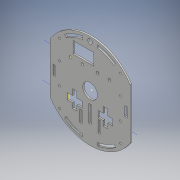
# Autodesk Inventor part: base_quick
Saved by Autodesk Inventor 2017.2 (Build 212233000, 233)
## iProperties
Created: 2017-07-13
Part Number: base_quick
Material: Generic
Document SubType Name: Modeling
Designer: Nic
Density: 1 g/cm^3
Appearance: Default
Author: Nic
Autodesk Inventor part; units mm, degrees
ref_plane "YZ Plane" through (0, 0, 0) normal (1, 0, 0) x (0, 1, 0)
ref_plane "XZ Plane" through (0, 0, 0) normal (0, 1, 0) x (-1, 0, 0)
ref_plane "XY Plane" through (0, 0, 0) normal (0, 0, 1) x (1, 0, 0)
sketch "Sketch1" plane through (0, 0, 0) normal (0, 1, 0) x (-1, 0, 0)
  line L0 (42.2, 26.8172) -> (42.2, -26.8172)
  line L1 (0, 0) -> (0, -50) construction
  line L2 (-42.2, 26.8172) -> (-42.2, -26.8172)
  arc A0 (42.2, 26.8172) -> (-42.2, 26.8172) centre (0, 0) ccw
  arc A1 (-42.2, -26.8172) -> (42.2, -26.8172) centre (0, 0) ccw
  line L3 (39.2, 5) -> (36.7, 5)
  line L4 (36.7, 5) -> (36.7, -5)
  line L5 (36.7, -5) -> (39.2, -5)
  line L6 (39.2, -5) -> (39.2, 5)
  circle A2 centre (0, 0) radius 7.75
  line L7 (1.25, -12) -> (-1.25, -12)
  line L8 (-1.25, -12) -> (-1.25, -30)
  line L9 (-1.25, -30) -> (1.25, -30)
  line L10 (1.25, -30) -> (1.25, -12)
  line L11 (10.95, -22) -> (8.45, -22)
  line L12 (8.45, -22) -> (8.45, -34)
  line L13 (8.45, -34) -> (10.95, -34)
  line L14 (10.95, -34) -> (10.95, -22)
  line L15 (8.45, -13.6) -> (8.45, -20)
  line L16 (24.05, -20) -> (24.05, -13.6)
  line L17 (18.55, -7.2) -> (13.95, -7.2)
  line L18 (13.95, -25.2) -> (18.55, -25.2)
  line L19 (18, 37.1) -> (-4, 37.1)
  line L20 (-4, 37.1) -> (-4, 24.85)
  line L21 (-4, 24.85) -> (18, 24.85)
  line L22 (18, 24.85) -> (18, 37.1)
  line L23 (25.2374, 36.0427) -> (26.9581, 38.5001)
  line L24 (0, 0) -> (7.6405, 43.3315) construction
  line L25 (7.6405, 43.3315) -> (8.1615, 46.286)
  line L26 (0, 0) -> (42.2, 0) construction
  line L27 (25.2374, -36.0427) -> (26.9581, -38.5001)
  line L28 (7.6405, -43.3315) -> (8.1615, -46.286)
  arc A3 (7.6405, -43.3315) -> (25.2374, -36.0427) centre (0, 0) ccw
  arc A4 (25.2374, 36.0427) -> (7.6405, 43.3315) centre (0, 0) ccw
  arc A5 (8.1615, -46.286) -> (26.9581, -38.5001) centre (0, 0) ccw
  arc A6 (26.9581, 38.5001) -> (8.1615, 46.286) centre (0, 0) ccw
  line L29 (0, 0) -> (25.2374, 36.0427) construction
  line L30 (16.25, -7.2) -> (16.25, -25.2) construction
  line L31 (18.55, -25.2) -> (18.55, -20)
  line L32 (18.55, -13.6) -> (18.55, -7.2)
  line L33 (24.05, -13.6) -> (18.55, -13.6)
  line L34 (13.95, -13.6) -> (8.45, -13.6)
  line L35 (13.95, -7.2) -> (13.95, -13.6)
  line L36 (13.95, -20) -> (13.95, -25.2)
  line L37 (8.45, -20) -> (13.95, -20)
  line L38 (18.55, -20) -> (24.05, -20)
  line L39 (-39.2, 5) -> (-36.7, 5)
  line L40 (-36.7, 5) -> (-36.7, -5)
  line L41 (-36.7, -5) -> (-39.2, -5)
  line L42 (-39.2, -5) -> (-39.2, 5)
  line L43 (-8.45, 16.1) -> (-8.45, 9.2)
  line L44 (-11.55, 9.2) -> (-11.55, 16.1)
  line L45 (-10.95, -22) -> (-8.45, -22)
  line L46 (-8.45, -22) -> (-8.45, -34)
  line L47 (-8.45, -34) -> (-10.95, -34)
  line L48 (-10.95, -34) -> (-10.95, -22)
  line L49 (-8.45, -13.6) -> (-8.45, -20)
  line L50 (-24.05, -20) -> (-24.05, -13.6)
  line L51 (-18.55, -7.2) -> (-13.95, -7.2)
  line L52 (-13.95, -25.2) -> (-18.55, -25.2)
  line L53 (-25.2374, 36.0427) -> (-26.9581, 38.5001)
  line L54 (-7.6405, 43.3315) -> (-8.1615, 46.286)
  line L55 (0, 0) -> (-42.2, 0) construction
  line L56 (-25.2374, -36.0427) -> (-26.9581, -38.5001)
  line L57 (-7.6405, -43.3315) -> (-8.1615, -46.286)
  arc A7 (-25.2374, -36.0427) -> (-7.6405, -43.3315) centre (0, 0) ccw
  arc A8 (-7.6405, 43.3315) -> (-25.2374, 36.0427) centre (0, 0) ccw
  arc A9 (-26.9581, -38.5001) -> (-8.1615, -46.286) centre (0, 0) ccw
  arc A10 (-8.1615, 46.286) -> (-26.9581, 38.5001) centre (0, 0) ccw
  line L58 (-18.55, -25.2) -> (-18.55, -20)
  line L59 (-18.55, -13.6) -> (-18.55, -7.2)
  line L60 (-24.05, -13.6) -> (-18.55, -13.6)
  line L61 (-13.95, -13.6) -> (-8.45, -13.6)
  line L62 (-13.95, -7.2) -> (-13.95, -13.6)
  line L63 (-13.95, -20) -> (-13.95, -25.2)
  line L64 (-8.45, -20) -> (-13.95, -20)
  line L65 (-18.55, -20) -> (-24.05, -20)
  circle A11 centre (0, 0) radius 45.5 construction
  circle A12 centre (32.2, -32.1467) radius 1
  circle A13 centre (32.2, 11.5) radius 1
  line L66 (11.95, 11.5) -> (32.2, 11.5) construction
  circle A14 centre (32.2, -11.5) radius 1
  circle A15 centre (32.2, 32.1467) radius 1
  circle A16 centre (-32.2, -32.1467) radius 1
  circle A17 centre (-32.2, 11.5) radius 1
  circle A18 centre (-32.2, -11.5) radius 1
  circle A19 centre (-32.2, 32.1467) radius 1
  arc A20 (-8.45, 16.1) -> (-11.55, 16.1) centre (-10, 16.1) ccw
  arc A21 (-11.55, 9.2) -> (-8.45, 9.2) centre (-10, 9.2) ccw
  arc A22 (-9.8689, 7.6556) -> (-8.45, 9.2) centre (-10, 9.2) ccw
  line L67 (11.55, 9.2) -> (11.55, 16.1)
  line L68 (8.45, 16.1) -> (8.45, 9.2)
  arc A23 (11.55, 16.1) -> (8.45, 16.1) centre (10, 16.1) ccw
  arc A24 (8.45, 9.2) -> (11.55, 9.2) centre (10, 9.2) ccw
  circle A25 centre (-8.05, 20.5) radius 1.4
  circle A26 centre (8.05, 20.5) radius 1.4
  circle A27 centre (-20.65, 20.5) radius 1.4
  circle A28 centre (20.65, 20.5) radius 1.4
  line L69 (-1.55, 11.2) -> (-1.55, 18.1)
  arc A29 (1.55, 18.1) -> (-1.55, 18.1) centre (0, 18.1) ccw
  line L70 (1.55, 18.1) -> (1.55, 11.2)
  arc A30 (-1.55, 11.2) -> (1.55, 11.2) centre (0, 11.2) ccw
  circle A31 centre (0, 45.5) radius 2.5
  line L71 (0, 45.5) -> (0, 50) construction
  line L72 (0, 50) -> (0, 45.5) construction
  point P0 (-16.25, -7.2)
  point P1 (26.0977, -37.2714)
  dimension "d1" = 42.2
  dimension "d2" = 50
  dimension "d5" = 10
  dimension "d6" = 35
  dimension "d7" = 44
  dimension "d8" = 47
  dimension "d9" = 10
  dimension "d10" = 3
  dimension "d11" = 2.5
  dimension "d12" = 15.5
  dimension "d13" = 12
  dimension "d14" = 18
  dimension "d15" = 1.25
  dimension "d20" = 12
  dimension "d21" = 10
  dimension "d22" = 12.25
  dimension "d23" = 4
  dimension "d24" = 22
  dimension "d26" = 4.6
  dimension "d27" = 6.4
  dimension "d28" = 18
  dimension "d30" = 5.5
  dimension "d39" = 10
  dimension "d40" = 2
  dimension "d47" = 20.25
  dimension "d52" = 2.8
  dimension "d55" = 12.6
  dimension "d57" = 20.5
  dimension "d58" = 3.1
  dimension "d59" = 6.9
  dimension "d60" = 3.1
  dimension "d61" = 11.2
  dimension "d62" = 13.1
  dimension "d63" = 16.1
  dimension "d64" = 2
  dimension "d65" = 6.5
  dimension "d66" = 24.85
  dimension "d67" = 5.2
  dimension "d68" = 25.2
  dimension "d69" = 5
  constraints: 146 end point, 49 symmetric about line, 39 point on circle, 32 centre point, 21 parallel, 8 coincident, 8 collinear, 8 horizontal, 8 perpendicular, 8 tangent, 5 equal radius, 5 vertical, 4 midpoint, 1 horizontal alignment, 1 point on line, 1 vertical alignment, 19 other
  measures "d1" distance between parallel lines of L1 L0
  measures "d2" radius of A1
  measures "d5" angle of L1 L25
  measures "d6" angle of L1 L23
  measures "d7" radius of A4
  measures "d8" radius of A6
  measures "d9" distance of L3.end L4.end
  measures "d10" distance between parallel lines of L0 L6
  measures "d11" distance of L4.end L5.end
  measures "d12" diameter of A2
  measures "d13" distance from line of point (0, 0) L7
  measures "d14" distance of L9.end L7.start
  measures "d15" distance between parallel lines of L10 L1
  measures "d20" distance of L13.end L11.start
  measures "d21" distance between parallel lines of L7 L11
  measures "d22" distance of L19.end L20.end
  measures "d23" distance between parallel lines of L1 L20
  measures "d24" distance of L19.start L19.end
  measures "d26" distance of L18.start L18.end
  measures "d27" distance of L16.start L16.end
  measures "d28" distance of L17.end L18.start
  measures "d30" distance between parallel lines of L15 L35
  measures "d39" distance from line of L0 A13.centre
  measures "d40" diameter of A12
  measures "d47" distance of L66.start L66.end
  measures "d52" diameter of A25
  measures "d55" distance of A28.centre A26.centre
  measures "d57" vertical distance of L1.start A26.centre
  measures "d58" distance between parallel lines of L43 L44
  measures "d59" distance of A21.centre A20.centre
  measures "d60" distance between parallel lines of L70 L69
  measures "d61" distance of point (0, 0) A30.centre
  measures "d62" distance between parallel lines of L44 L70
  measures "d63" distance of A25.centre A26.centre
  measures "d64" vertical distance of A29.centre A23.centre
  measures "d65" distance from line of A13.centre L3
  measures "d66" distance from line of point (0, 0) L21
  measures "d67" distance between parallel lines of L38 L18
  measures "d68" distance between parallel lines of L18 L26
  measures "d69" diameter of A31
extrude "Extrusion1" add sketch "Sketch1" along normal blind 1.5 contours L0 A1 L2 A0 | L43 A21 L44 A20 | A24 L68 A23 L67 | L69 A29 L70 A30
sketch "Sketch2" plane through (0, 1.5, 0) normal (0, 1, 0) x (1, 0, 0)
  line L0 (-24.05, 13.6) -> (-24.05, 20) construction
  line L1 (24.05, 13.6) -> (24.05, 20) construction
  line L2 (24.05, 16.8) -> (49.05, 16.8) construction
  line L3 (-24.05, 16.8) -> (-24.05, -20.5) construction
  line L4 (-24.05, -20.5) -> (-49.8842, -20.5) construction
  circle A0 centre (-20.65, -20.5) radius 1.4 projected
  line L5 (-24.05, 20) -> (-24.05, 13.6) projected
  line L6 (-24.05, 16.8) -> (-50.8471, 16.8) construction
  point P0 (0, 0)
  constraints: 8 end point, 3 horizontal, 2 midpoint, 1 point on line, 1 vertical
body "Solid1"
